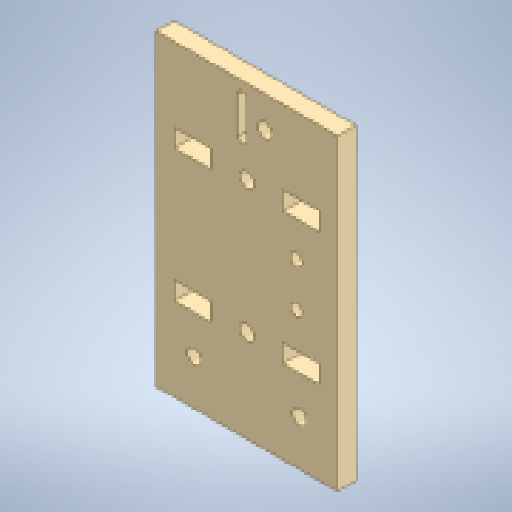
# Autodesk Inventor part: дно_каретки
Saved by Autodesk Inventor 2024 (Build 280153000, 153)
## iProperties
Created: 2026-02-03
Part Number: дно_каретки
Material: Типовые
Document SubType Name: Modeling
Designer: DELL
Density: 1 g/cm^3
Appearance: Пшеничный
Author: DELL
Autodesk Inventor part; units mm, degrees
ref_plane "YZ Plane" through (0, 0, 0) normal (1, 0, 0) x (0, 1, 0)
ref_plane "XZ Plane" through (0, 0, 0) normal (0, 1, 0) x (-1, 0, 0)
ref_plane "XY Plane" through (0, 0, 0) normal (0, 0, 1) x (1, 0, 0)
sketch "Эскиз1" plane through (0, 0, 0) normal (0, 0, 1) x (1, 0, 0)
  line L0 (-26.5, -35) -> (13.5, -35)
  line L1 (13.5, -35) -> (13.5, 33)
  line L2 (13.5, 33) -> (-26.5, 33)
  line L3 (-26.5, 33) -> (-26.5, -35)
  line L4 (-22.5, -16.6) -> (-14.5, -16.6)
  line L5 (-14.5, -16.6) -> (-14.5, -12.6)
  line L6 (-14.5, -12.6) -> (-22.5, -12.6)
  line L7 (-22.5, -12.6) -> (-22.5, -16.6)
  line L8 (1.5, -16.6) -> (9.5, -16.6)
  line L9 (9.5, -16.6) -> (9.5, -12.6)
  line L10 (9.5, -12.6) -> (1.5, -12.6)
  line L11 (1.5, -12.6) -> (1.5, -16.6)
  line L12 (-22.5, 16.6) -> (-14.5, 16.6)
  line L13 (-14.5, 16.6) -> (-14.5, 12.6)
  line L14 (-14.5, 12.6) -> (-22.5, 12.6)
  line L15 (-22.5, 12.6) -> (-22.5, 16.6)
  line L16 (1.5, 12.6) -> (9.5, 12.6)
  line L17 (9.5, 12.6) -> (9.5, 16.6)
  line L18 (9.5, 16.6) -> (1.5, 16.6)
  line L19 (1.5, 16.6) -> (1.5, 12.6)
  line L20 (-18.5, -12.6) -> (-18.5, -3.7782) construction
  line L21 (5.5, -12.6) -> (5.5, -5.4201) construction
  point P0 (0, 0)
  point P1 (-14.5, -14.6)
  point P2 (1.5, -14.6)
  point P3 (5.5, 12.6)
  point P4 (-18.5, 12.6)
  dimension "d0" = 68
  dimension "d1" = 40
  dimension "d2" = 8
  dimension "d3" = 4
  dimension "d5" = 4
  dimension "d10" = 8
  dimension "d12" = 4
  dimension "d13" = 16
  dimension "d32" = 8
  dimension "d33" = 4
  dimension "d34" = 8
  dimension "d35" = 25.2
  dimension "d54" = 16.4
  dimension "d55" = 25.2
  constraints: 44 end point, 10 parallel, 6 midpoint, 5 horizontal, 5 perpendicular, 4 point on line, 2 vertical
  measures "d0" distance of L0.end L1.end
  measures "d1" distance of L1.end L2.end
  measures "d2" distance of L6.end L5.end
  measures "d3" distance of L5.end L4.end
  measures "d5" distance between parallel lines of L3 L7
  measures "d10" distance of L10.end L9.end
  measures "d12" distance of L8.end L9.end
  measures "d13" distance of point (-14.5, -14.6) point (1.5, -14.6)
  measures "d32" distance of L13.end L14.end
  measures "d33" distance of L12.end L13.end
  measures "d34" distance of L18.end L17.end
  measures "d35" distance between parallel lines of L16 L10
  measures "d54" distance between parallel lines of L2 L18
  measures "d55" distance between parallel lines of L14 L6
extrude "Выдавливание1" add sketch "Эскиз1" along normal blind 4
sketch "Эскиз3" plane through (0, 0, 4) normal (0, 0, 1) x (1, 0, 0)
  line L0 (1.5, -16.6) -> (1.5, -12.6) projected
  line L1 (-14.5, -12.6) -> (-14.5, -16.6) projected
  circle A0 centre (-6.5, 14.6) radius 1.6
  circle A1 centre (-6.5, -14.6) radius 1.6
  line L2 (-14.5, 14.6) -> (1.5, 14.6)
  line L3 (-14.5, -14.6) -> (1.5, -14.6)
  line L4 (-14.5, 16.6) -> (-14.5, 12.6) projected
  line L5 (1.5, 12.6) -> (1.5, 16.6) projected
  point P0 (0, 0)
  point P1 (-14.5, 14.6)
  point P2 (1.5, 14.6)
  dimension "d27" = 3.2
  dimension "d28" = 3.2
  constraints: 7 midpoint, 4 end point, 2 centre point, 2 coincident, 1 point on line
  measures "d27" diameter of A0
  measures "d28" diameter of A1
extrude "Выдавливание3" cut sketch "Эскиз3" against normal blind 4
sketch "Эскиз4" plane through (0, 0, 0) normal (0, 0, -1) x (-1, 0, 0)
  line L0 (-25.5, 33) -> (9.5, 33) construction
  line L1 (9.5, 33) -> (9.5, 19) construction
  line L2 (9.5, 19) -> (-25.5, 19) construction
  line L3 (-25.5, 19) -> (-25.5, 33) construction
  line L4 (-13.5, 33) -> (26.5, 33) projected
  line L5 (-13.5, -35) -> (-13.5, 33) projected
  circle A0 centre (2.5, 26) radius 1.6
  line L6 (7.5, 21) -> (7.5, 31) construction
  line L7 (8.5, 22) -> (8.5, 30)
  line L8 (6.5, 30) -> (6.5, 22)
  arc A1 (6.5, 22) -> (8.5, 22) centre (7.5, 22) ccw
  arc A2 (8.5, 30) -> (6.5, 30) centre (7.5, 30) ccw
  line L9 (9.5, 26) -> (-1.5724, 26)
  point P0 (0, 0)
  point P1 (-8, 33)
  point P2 (-25.5, 26)
  point P3 (7.5, 26)
  dimension "d39" = 35
  dimension "d40" = 14
  dimension "d41" = 12
  dimension "d42" = 3.2
  dimension "d43" = 7
  dimension "d44" = 10
  dimension "d45" = 2
  dimension "d46" = 5
  constraints: 18 end point, 6 point on circle, 5 point on line, 4 midpoint, 4 tangent, 3 centre point, 3 parallel, 2 horizontal, 1 perpendicular, 1 vertical
  measures "d39" distance of L1.end L2.end
  measures "d40" distance of L0.end L1.end
  measures "d41" distance from line of L5 point (-25.5, 26)
  measures "d42" diameter of A0
  measures "d43" distance of A0.centre L9.start
  measures "d44" distance of L6.start L6.end
  measures "d45" diameter of A2
  measures "d46" distance of point (7.5, 26) A0.centre
extrude "Выдавливание4" cut sketch "Эскиз4" against normal blind 4
sketch "Эскиз5" plane through (0, 0, 4) normal (0, 0, 1) x (1, 0, 0)
  line L0 (4.3225, 4.75) -> (4.3225, -4.75)
  line L1 (0, 0) -> (13.5, 0) construction
  line L2 (13.5, -35) -> (13.5, 33) construction
  circle A0 centre (4.3225, 4.75) radius 1.3
  circle A1 centre (4.3225, -4.75) radius 1.3
  point P0 (4.3225, 0)
  dimension "d49" = 9.5
  dimension "d50" = 2.6
  dimension "d51" = 2.6
  constraints: 4 end point, 2 centre point, 2 coincident, 2 point on line, 1 horizontal, 1 midpoint, 1 vertical
  measures "d49" distance of L0.start L0.end
  measures "d50" diameter of A0
  measures "d51" diameter of A1
extrude "Выдавливание5" cut sketch "Эскиз5" against normal blind 4
sketch "Эскиз7" plane through (0, 0, 4) normal (0, 0, 1) x (1, 0, 0)
  line L0 (23.5, -19) -> (23.5, -23) construction
  line L1 (-19.8, -23) -> (-19.8, -27) construction
  line L2 (-19.8, -27) -> (-36.5, -27) construction
  line L3 (-36.5, -27) -> (-36.5, -23) construction
  line L4 (-36.5, -23) -> (-19.8, -23) construction
  line L5 (3.5, -23) -> (3.5, -27) construction
  line L6 (3.5, -27) -> (-16.5, -27) construction
  line L7 (-16.5, -27) -> (-16.5, -23) construction
  line L8 (-16.5, -23) -> (3.5, -23) construction
  line L9 (6.8, -27) -> (6.8, -23) construction
  line L10 (6.8, -23) -> (23.5, -23) construction
  line L11 (23.5, -23) -> (23.5, -27) construction
  line L12 (23.5, -27) -> (6.8, -27) construction
  line L13 (-19.8, -27) -> (-16.5, -23) construction
  line L14 (3.5, -27) -> (6.8, -23) construction
  circle A0 centre (-18.15, -25) radius 1.6
  circle A1 centre (5.15, -25) radius 1.6
  dimension "d60" = 3.2
  dimension "d61" = 3.2
  constraints: 30 end point, 7 vertical, 6 horizontal, 2 centre point, 2 midpoint, 1 parallel, 13 other
  measures "d60" diameter of A0
  measures "d61" diameter of A1
extrude "Выдавливание6" cut sketch "Эскиз7" against normal blind 10
